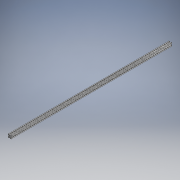
# Autodesk Inventor part: Alumunium Profile 20 x 20
Saved by Autodesk Inventor 2022 (Build 260153000, 153)
## iProperties
Created: 2022-03-03
Part Number: Alumunium Profile 20 x 20
Material: Aluminum 6061
Document SubType Name: Modeling
Designer: ASUS
Density: 2.7 g/cm^3
Appearance: Aluminum - Polished
Author: ASUS
Autodesk Inventor part; units mm, degrees
ref_plane "YZ Plane" through (0, 0, 0) normal (1, 0, 0) x (0, 1, 0)
ref_plane "XZ Plane" through (0, 0, 0) normal (0, 1, 0) x (-1, 0, 0)
ref_plane "XY Plane" through (0, 0, 0) normal (0, 0, 1) x (1, 0, 0)
sketch "Sketch1" plane through (0, 0, 0) normal (0, 0, 1) x (1, 0, 0)
  circle A0 centre (10.0217, 10.0217) radius 2.5
  line L0 (7.4217, 6.0217) -> (12.6217, 6.0217)
  line L1 (14.0217, 7.4217) -> (14.0217, 12.6217)
  line L2 (12.6217, 14.0217) -> (7.4217, 14.0217)
  line L3 (6.0217, 12.6217) -> (6.0217, 7.4217)
  line L4 (1.5217, 20.0217) -> (6.4217, 20.0217)
  line L5 (18.5217, 20.0217) -> (13.6217, 20.0217)
  arc A1 (20.0217, 18.5217) -> (18.5217, 20.0217) centre (18.5217, 18.5217) ccw
  line L6 (6.9217, 19.5217) -> (6.4217, 19.5217)
  line L7 (6.4217, 19.5217) -> (6.4217, 20.0217)
  line L8 (13.1217, 19.5217) -> (13.6217, 19.5217)
  line L9 (13.6217, 19.5217) -> (13.6217, 20.0217)
  line L10 (0.0217, 18.5217) -> (0.0217, 13.6217)
  arc A2 (1.5217, 20.0217) -> (0.0217, 18.5217) centre (1.5217, 18.5217) ccw
  line L11 (20.0217, 18.5217) -> (20.0217, 13.6217)
  line L12 (0.0217, 1.5217) -> (0.0217, 6.4217)
  arc A3 (0.0217, 1.5217) -> (1.5217, 0.0217) centre (1.5217, 1.5217) ccw
  line L13 (20.0217, 1.5217) -> (20.0217, 6.4217)
  line L14 (1.5217, 0.0217) -> (6.4217, 0.0217)
  line L15 (18.5217, 0.0217) -> (13.6217, 0.0217)
  arc A4 (18.5217, 0.0217) -> (20.0217, 1.5217) centre (18.5217, 1.5217) ccw
  line L16 (0.0217, 13.6217) -> (0.5217, 13.6217)
  line L17 (0.5217, 13.6217) -> (0.5217, 13.1217)
  line L18 (0.0217, 6.4217) -> (0.5217, 6.4217)
  line L19 (0.5217, 6.4217) -> (0.5217, 6.9217)
  line L20 (20.0217, 6.4217) -> (19.5217, 6.4217)
  line L21 (19.5217, 6.4217) -> (19.5217, 6.9217)
  line L22 (20.0217, 13.6217) -> (19.5217, 13.6217)
  line L23 (19.5217, 13.6217) -> (19.5217, 13.1217)
  line L24 (6.9217, 0.5217) -> (6.4217, 0.5217)
  line L25 (6.4217, 0.5217) -> (6.4217, 0.0217)
  line L26 (13.1217, 0.5217) -> (13.6217, 0.5217)
  line L27 (13.6217, 0.5217) -> (13.6217, 0.0217)
  line L28 (0.5217, 6.9217) -> (2.0217, 6.9217)
  line L29 (6.9217, 0.5217) -> (6.9217, 2.0217)
  line L30 (6.9217, 2.0217) -> (4.6288, 2.0217)
  arc A5 (4.2753, 2.8753) -> (4.6288, 2.0217) centre (4.6288, 2.5217) ccw
  line L31 (2.0217, 4.6288) -> (2.0217, 6.9217)
  arc A6 (2.0217, 4.6288) -> (2.8753, 4.2753) centre (2.5217, 4.6288) ccw
  line L32 (2.8753, 4.2753) -> (6.0217, 7.4217)
  line L33 (4.2753, 2.8753) -> (7.4217, 6.0217)
  line L34 (13.1217, 0.5217) -> (13.1217, 2.0217)
  line L35 (13.1217, 2.0217) -> (15.4146, 2.0217)
  line L36 (18.0217, 4.6288) -> (18.0217, 6.9217)
  arc A7 (17.1682, 4.2753) -> (18.0217, 4.6288) centre (17.5217, 4.6288) ccw
  line L37 (18.0217, 6.9217) -> (19.5217, 6.9217)
  line L38 (13.1217, 19.5217) -> (13.1217, 18.0217)
  line L39 (13.1217, 18.0217) -> (15.4146, 18.0217)
  arc A8 (15.7682, 17.1682) -> (15.4146, 18.0217) centre (15.4146, 17.5217) ccw
  line L40 (18.0217, 15.4146) -> (18.0217, 13.1217)
  arc A9 (18.0217, 15.4146) -> (17.1682, 15.7682) centre (17.5217, 15.4146) ccw
  line L41 (18.0217, 13.1217) -> (19.5217, 13.1217)
  line L42 (6.9217, 19.5217) -> (6.9217, 18.0217)
  line L43 (6.9217, 18.0217) -> (4.6288, 18.0217)
  line L44 (2.0217, 15.4146) -> (2.0217, 13.1217)
  arc A10 (2.8753, 15.7682) -> (2.0217, 15.4146) centre (2.5217, 15.4146) ccw
  line L45 (2.0217, 13.1217) -> (0.5217, 13.1217)
  line L46 (12.6217, 6.0217) -> (15.7682, 2.8753)
  arc A11 (15.4146, 2.0217) -> (15.7682, 2.8753) centre (15.4146, 2.5217) ccw
  line L47 (14.0217, 7.4217) -> (17.1682, 4.2753)
  line L48 (12.6217, 14.0217) -> (15.7682, 17.1682)
  line L49 (14.0217, 12.6217) -> (17.1682, 15.7682)
  line L50 (6.0217, 12.6217) -> (2.8753, 15.7682)
  line L51 (7.4217, 14.0217) -> (4.2753, 17.1682)
  arc A12 (4.6288, 18.0217) -> (4.2753, 17.1682) centre (4.6288, 17.5217) ccw
  point P0 (0, 0)
  constraints: 104 end point, 24 point on circle, 13 centre point
extrude "Extrusion1" add sketch "Sketch1" against normal blind 1000
body "Solid1"
